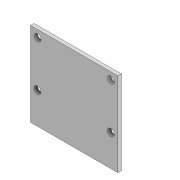
# Autodesk Inventor part: raspberry pi camera v2
Saved by Autodesk Inventor 2022 (Build 260153000, 153)
## iProperties
Created: 2024-06-26
Part Number: raspberry pi camera v2
Material: Generic
Document SubType Name: Modeling
Designer: david
Density: 1 g/cm^3
Appearance: Default
Author: david
Autodesk Inventor part; units mm, degrees
ref_plane "YZ Plane" through (0, 0, 0) normal (1, 0, 0) x (0, 1, 0)
ref_plane "XZ Plane" through (0, 0, 0) normal (0, 1, 0) x (-1, 0, 0)
ref_plane "XY Plane" through (0, 0, 0) normal (0, 0, 1) x (1, 0, 0)
sketch "Sketch1" plane through (0, 0, 0) normal (0, 0, 1) x (1, 0, 0)
  line L0 (12.5, -12) -> (-12.5, -12)
  line L1 (-12.5, -12) -> (-12.5, 12)
  line L2 (-12.5, 12) -> (12.5, 12)
  line L3 (12.5, 12) -> (12.5, -12)
  line L4 (12.5, -12) -> (-12.5, 12) construction
  line L5 (-12.5, -12) -> (12.5, 12) construction
  point P0 (0, 0)
  dimension "d0" = 24
  dimension "d1" = 25
  constraints: 12 end point, 2 midpoint, 2 parallel, 1 horizontal, 1 perpendicular
  measures "d0" distance of L0.end L1.end
  measures "d1" distance of L0.start L0.end
extrude "Extrusion1" add sketch "Sketch1" along normal mid plane 1
sketch "Sketch2" plane through (0, 0, -0.5) normal (0, 0, -1) x (-1, 0, 0)
  line L0 (-5.5, 3.5) -> (5.5, 3.5)
  line L1 (5.5, 3.5) -> (5.5, -7.5)
  line L2 (5.5, -7.5) -> (-5.5, -7.5)
  line L3 (-5.5, -7.5) -> (-5.5, 3.5)
  line L4 (-5.5, 3.5) -> (5.5, -7.5) construction
  line L5 (5.5, 3.5) -> (-5.5, -7.5) construction
  line L6 (-12.5, -12) -> (12.5, -12) projected
  point P0 (0, 0)
  point P1 (0, -2)
  point P2 (0, -2)
  dimension "d4" = 11
  dimension "d5" = 11
  dimension "d6" = 4.5
  constraints: 12 end point, 3 midpoint, 2 parallel, 1 horizontal, 1 perpendicular, 1 vertical alignment
  measures "d4" distance of L1.end L2.end
  measures "d5" distance of L0.end L1.end
  measures "d6" distance between parallel lines of L6 L2
extrude "Extrusion2" add sketch "Sketch2" along normal blind 5
sketch "Sketch3" plane through (0, 0, -0.5) normal (0, 0, -1) x (-1, 0, 0)
  circle A0 centre (0, -2) radius 4.5
  line L0 (5.5, 3.5) -> (-5.5, 3.5) projected
  line L1 (5.5, -7.5) -> (5.5, 3.5) projected
  point P0 (0, 0)
  point P1 (0, 3.5)
  point P2 (5.5, -2)
  dimension "d9" = 9
  constraints: 2 midpoint, 1 centre point, 1 horizontal alignment, 1 vertical alignment
  measures "d9" diameter of A0
extrude "Extrusion3" add sketch "Sketch3" along normal blind 8
sketch "Sketch4" plane through (0, 0, -0.5) normal (0, 0, -1) x (-1, 0, 0)
  line L0 (3, 6) -> (-5.5, 6)
  line L1 (-5.5, 6) -> (-5.5, 10)
  line L2 (-5.5, 10) -> (3, 10)
  line L3 (3, 10) -> (3, 6)
  line L4 (3, 6) -> (-5.5, 10) construction
  line L5 (-5.5, 6) -> (3, 10) construction
  line L6 (12.5, 12) -> (-12.5, 12) projected
  line L7 (-12.5, 12) -> (-12.5, -12) projected
  point P0 (0, 0)
  point P1 (-1.25, 8)
  dimension "d12" = 8.5
  dimension "d13" = 4
  dimension "d14" = 2
  dimension "d15" = 7
  constraints: 12 end point, 2 midpoint, 2 parallel, 1 horizontal, 1 perpendicular
  measures "d12" distance of L1.end L2.end
  measures "d13" distance of L0.end L1.end
  measures "d14" distance between parallel lines of L6 L2
  measures "d15" distance between parallel lines of L1 L7
extrude "Extrusion4" add sketch "Sketch4" along normal blind 1.5
sketch "Sketch5" plane through (0, 0, -0.5) normal (0, 0, -1) x (-1, 0, 0)
  line L0 (11.5, -4) -> (-11.5, -4) construction
  line L1 (-11.5, -4) -> (-11.5, 11) construction
  line L2 (-11.5, 11) -> (11.5, 11) construction
  line L3 (11.5, 11) -> (11.5, -4) construction
  line L4 (11.5, -4) -> (-11.5, 11) construction
  line L5 (-11.5, -4) -> (11.5, 11) construction
  line L6 (12.5, 12) -> (-12.5, 12) projected
  line L7 (12.5, -12) -> (12.5, 12) projected
  circle A0 centre (-10.5, 10) radius 1
  circle A1 centre (10.5, 10) radius 1
  circle A2 centre (-10.5, -3) radius 1
  circle A3 centre (10.5, -3) radius 1
  point P0 (0, 0)
  point P1 (0, 3.5)
  point P2 (0, 11)
  point P3 (0, 12)
  dimension "d19" = 15
  dimension "d20" = 1
  dimension "d21" = 1
  dimension "d22" = 2
  dimension "d23" = 2
  dimension "d24" = 2
  dimension "d25" = 2
  constraints: 12 end point, 8 tangent, 4 centre point, 4 midpoint, 2 parallel, 1 horizontal, 1 perpendicular, 1 vertical alignment
  measures "d19" distance between parallel lines of L0 L2
  measures "d20" distance between parallel lines of L6 L2
  measures "d21" distance between parallel lines of L7 L3
  measures "d22" diameter of A0
  measures "d23" diameter of A1
  measures "d24" diameter of A2
  measures "d25" diameter of A3
extrude "Extrusion5" cut sketch "Sketch5" against normal through all
equation "\"d5\" = d4"
equation "\"d23\" = d22"
equation "\"d24\" = d22"
equation "\"d25\" = d24"
body "Solid1"
